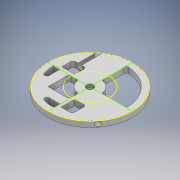
# Autodesk Inventor part: servoPlate
Saved by Autodesk Inventor 2018 (Build 220112000, 112)
## iProperties
Created: 2020-03-23
Part Number: servoPlate
Material: Generic
Document SubType Name: Modeling
Designer: technik
Density: 1 g/cm^3
Appearance: Default
Mass: 16.1735 g
Surface Area: 95.1977 cm^2
Volume: 16.1735 cm^3
Author: technik
Autodesk Inventor part; units mm, degrees
ref_plane "YZ Plane" through (0, 0, 0) normal (1, 0, 0) x (0, 1, 0)
ref_plane "XZ Plane" through (0, 0, 0) normal (0, 1, 0) x (-1, 0, 0)
ref_plane "XY Plane" through (0, 0, 0) normal (0, 0, 1) x (1, 0, 0)
sketch "Sketch1" plane through (0, 0, 0) normal (0, 0, 1) x (1, 0, 0)
  circle A0 centre (0, 0) radius 37
  dimension "d0" = 74
  constraints: 1 centre point, 1 coincident
  measures "d0" diameter of A0
extrude "Extrusion1" add sketch "Sketch1" along normal blind 5
sketch "Sketch2" plane through (0, 0, 5) normal (0, 0, 1) x (1, 0, 0)
  circle A0 centre (0, 0) radius 3
  dimension "d3" = 6
  constraints: 1 centre point, 1 coincident
  measures "d3" diameter of A0
extrude "Extrusion2" cut sketch "Sketch2" against normal blind 3
sketch "Sketch5" plane through (0, 0, 2) normal (0, 0, 1) x (1, 0, 0)
  circle A0 centre (0, 0) radius 1.75
  dimension "d6" = 3.5
  constraints: 1 centre point, 1 coincident
  measures "d6" diameter of A0
extrude "Extrusion3" cut sketch "Sketch5" along normal through all both and the other way through all
sketch "Sketch6" plane through (0, 0, 5) normal (0, 0, 1) x (1, 0, 0)
  circle A0 centre (0, 0) radius 37 projected
  line L0 (0, 37) -> (0, -37)
  line L1 (-37, 0) -> (37, 0)
  constraints: 4 end point, 4 point on circle, 1 perpendicular, 1 vertical
sketch "Sketch12" plane through (0, 0, 5) normal (0, 0, 1) x (1, 0, 0)
  ellipse E0 centre (-0.0097, 0.019) end of major axis (15.8068, 5.5327) minor radius 16.75 projected
  point P0 (0, 0)
  constraints: 1 other
sketch "Sketch13" plane through (0, 0, 5) normal (0, 0, 1) x (1, 0, 0)
  ellipse E0 centre (6.7485, -22.3457) end of major axis (6.7485, -16.3457) minor radius 0.0028 (6.7485, -28.3457) -> (6.7485, -16.3457) ccw
  line L0 (6.7485, -16.3457) -> (6.756, -16.3457)
  ellipse E1 centre (6.756, -17.3457) end of major axis (6.756, -16.3457) minor radius 0.0005 (6.7565, -17.3457) -> (6.756, -16.3457) ccw
  line L1 (6.7565, -17.3457) -> (6.7565, -27.3457)
  ellipse E2 centre (6.756, -27.3457) end of major axis (6.756, -26.3457) minor radius 0.0005 (6.756, -28.3457) -> (6.7565, -27.3457) ccw
  line L2 (6.756, -28.3457) -> (6.7485, -28.3457)
  line L3 (2.7586, -17.3457) -> (2.7586, -27.3457)
  line L4 (4.7586, -27.3457) -> (4.7586, -17.3457)
  ellipse E3 centre (2.744, -17.3457) end of major axis (2.744, -16.3457) minor radius 0.0005 (2.744, -16.3457) -> (2.7435, -17.3457) ccw
  line L5 (2.7435, -17.3457) -> (2.7435, -27.3457)
  ellipse E4 centre (2.744, -27.3457) end of major axis (2.744, -26.3457) minor radius 0.0005 (2.7435, -27.3457) -> (2.744, -28.3457) ccw
  line L6 (2.744, -28.3457) -> (2.7461, -28.3457)
  ellipse E5 centre (2.7461, -27.3457) end of major axis (2.7461, -26.3457) minor radius 0.0005 (2.7456, -27.3457) -> (2.7461, -28.3457) ccw
  line L7 (2.7456, -17.3457) -> (2.7456, -27.3457)
  ellipse E6 centre (2.7461, -17.3457) end of major axis (2.7461, -16.3457) minor radius 0.0005 (2.7461, -16.3457) -> (2.7456, -17.3457) ccw
  line L8 (2.7461, -16.3457) -> (2.744, -16.3457)
  ellipse E7 centre (2.7442, -22.3457) end of major axis (2.7442, -21.3457) minor radius 0.0005
  ellipse E8 centre (-21.634, 6.7452) end of major axis (-27.634, 6.7452) minor radius 0.0082 (-27.634, 6.7452) -> (-15.634, 6.7452) ccw
  line L9 (-27.634, 6.7452) -> (-27.634, 6.7234)
  ellipse E9 centre (-26.634, 6.7234) end of major axis (-27.634, 6.7234) minor radius 0.0014 (-27.634, 6.7234) -> (-26.634, 6.7221) ccw
  line L10 (-26.634, 6.7221) -> (-16.634, 6.722)
  ellipse E10 centre (-16.634, 6.7234) end of major axis (-17.634, 6.7234) minor radius 0.0014 (-16.634, 6.722) -> (-15.634, 6.7234) ccw
  line L11 (-15.634, 6.7234) -> (-15.634, 6.7452)
  ellipse E11 centre (-21.634, 4.7574) end of major axis (-22.634, 4.7574) minor radius 0.0014
  ellipse E12 centre (-26.634, 4.7581) end of major axis (-25.634, 4.7581) minor radius 0.0014 (-26.634, 4.7594) -> (-27.634, 4.7581) ccw
  line L12 (-27.634, 4.7581) -> (-27.634, 4.752)
  ellipse E13 centre (-26.634, 4.752) end of major axis (-25.634, 4.752) minor radius 0.0014 (-26.634, 4.7533) -> (-27.634, 4.752) ccw
  line L13 (-16.634, 4.7533) -> (-26.634, 4.7533)
  ellipse E14 centre (-16.634, 4.752) end of major axis (-15.634, 4.752) minor radius 0.0014 (-15.634, 4.752) -> (-16.634, 4.7533) ccw
  line L14 (-15.634, 4.752) -> (-15.634, 4.7581)
  ellipse E15 centre (-16.634, 4.7581) end of major axis (-15.634, 4.7581) minor radius 0.0014 (-15.634, 4.7581) -> (-16.634, 4.7594) ccw
  line L15 (-16.634, 4.7594) -> (-26.634, 4.7594)
  ellipse E16 centre (-26.634, 2.7581) end of major axis (-27.634, 2.7581) minor radius 0.0014 (-26.634, 2.7594) -> (-27.634, 2.7581) ccw
  line L16 (-26.634, 2.7594) -> (-16.634, 2.7594)
  ellipse E17 centre (-16.634, 2.7581) end of major axis (-17.634, 2.7581) minor radius 0.0014 (-15.634, 2.7581) -> (-16.634, 2.7594) ccw
  line L17 (-15.634, 2.7581) -> (-15.634, 2.752)
  ellipse E18 centre (-16.634, 2.752) end of major axis (-17.634, 2.752) minor radius 0.0014 (-15.634, 2.752) -> (-16.634, 2.7533) ccw
  line L18 (-26.634, 2.7533) -> (-16.634, 2.7533)
  ellipse E19 centre (-26.634, 2.752) end of major axis (-27.634, 2.752) minor radius 0.0014 (-26.634, 2.7533) -> (-27.634, 2.752) ccw
  line L19 (-27.634, 2.752) -> (-27.634, 2.7581)
  ellipse E20 centre (-21.634, 2.7574) end of major axis (-22.634, 2.7574) minor radius 0.0014
  line L20 (2.7461, -28.3457) -> (4.7586, -28.3457)
  line L21 (4.7586, -28.3457) -> (4.7586, -16.3457)
  line L22 (4.7586, -16.3457) -> (2.7461, -16.3457)
  line L23 (2.7461, -16.3457) -> (2.7461, -28.3457)
  line L24 (4.7586, -28.3457) -> (12.7435, -28.3457)
  line L25 (12.7435, -28.3457) -> (12.7435, -16.3457)
  line L26 (12.7435, -16.3457) -> (4.7586, -16.3457)
  line L27 (4.7586, -16.3457) -> (4.7586, -28.3457)
  line L28 (-27.634, 2.752) -> (-16.1272, 2.752)
  line L29 (-16.1272, 2.752) -> (-16.1272, 12.752)
  line L30 (-16.1272, 12.752) -> (-27.634, 12.752)
  line L31 (-27.634, 12.752) -> (-27.634, 2.752)
  point P0 (0, 0)
extrude "Extrusion9" cut sketch "Sketch13" against normal through all contours L24 L21 L4 L26 E0 | E7 | E2 L1 E1 L26 L25 L24 | L20 E4 L5 E3 L22 L21 L4 | L31 L30 L29 E8 | E8 L29 E10 L10 E9 L9 | E9 L10 E10 L29 E15 L15 E12 L31 | E12 L15 E15 L29 E14 L13 E13 L12 | E13 L13 E14 L29 E17 L16 E16 L31 | L29 E18 L18 L16 E17
sketch "Sketch14" plane through (0, 0, 5) normal (0, 0, 1) x (1, 0, 0)
  line L0 (12.7435, -16.3457) -> (12.7435, -28.3457) projected
  line L1 (2.7461, -28.3457) -> (2.7461, -16.3457) projected
  line L2 (12.7435, -16.3457) -> (2.7461, -16.3457)
  line L3 (2.7461, -16.3457) -> (2.7461, -28.3457)
  line L4 (2.7461, -28.3457) -> (12.7435, -28.3457)
  line L5 (12.7435, -28.3457) -> (12.7435, -16.3457)
  point P0 (0, 0)
  constraints: 8 end point, 2 parallel, 1 horizontal, 1 perpendicular
extrude "Extrusion10" cut sketch "Sketch14" against normal through all
sketch "Sketch17" plane through (2.7461, -28.3457, 5) normal (1, 0, 0) x (0, 0, -1)
  ellipse E0 centre (2.2619, 6) end of major axis (2.2619, 7) minor radius 1 projected
  circle A0 centre (2.2619, 6) radius 2
  point P0 (5, 28.3457)
  dimension "d47" = 4
  constraints: 1 centre point, 1 coincident, 1 other
  measures "d47" diameter of A0
extrude "Extrusion12" cut sketch "Sketch17" along normal through all contours E0 | A0
sketch "Sketch19" plane through (-27.634, 2.752, 5) normal (0, 1, 0) x (1, 0, 0)
  ellipse E0 centre (6, 1.9244) end of major axis (5, 1.924) minor radius 1 projected
  circle A0 centre (6, 1.9244) radius 2.5
  point P0 (27.634, 5)
  dimension "d52" = 5
  constraints: 1 centre point, 1 coincident, 1 other
  measures "d52" diameter of A0
extrude "Extrusion14" cut sketch "Sketch19" along normal through all contours E0 | A0
sketch "Sketch20" plane through (0, 0, 5) normal (0, 0, 1) x (1, 0, 0)
  circle A0 centre (0, 0) radius 1.75 projected
  circle A1 centre (0, 0) radius 37
  line L0 (0, 0) -> (1.75, 0)
  line L1 (10, 0) -> (32, 0)
  line L2 (0, 0) -> (0, 1.75)
  line L3 (0, 10) -> (0, 32)
  line L4 (0, 0) -> (-1.75, 0)
  line L5 (-10, 0) -> (-32, 0)
  line L6 (0, 0) -> (0, -1.75)
  line L7 (0, -10) -> (0, -32)
  arc A2 (32, 0) -> (0, 32) centre (0, 0) ccw
  arc A3 (-32, 0) -> (0, -32) centre (0, 0) ccw
  arc A4 (-10, 0) -> (0, -10) centre (0, 0) ccw
  arc A5 (10, 0) -> (0, 10) centre (0, 0) ccw
  constraints: 16 end point, 12 point on circle, 8 perpendicular, 5 centre point, 2 coincident, 2 horizontal, 2 vertical
extrude "Extrusion15" cut sketch "Sketch20" against normal blind 10 contours A5 L3 A2 L1 | A4 L7 A3 L5
sketch "Sketch21" plane through (0, 0, 5) normal (0, 0, 1) x (1, 0, 0)
  line L0 (-32, 0) -> (-10, 0) projected
  line L1 (-18.4966, 0) -> (-26.4966, 0)
  line L2 (-26.4966, 0) -> (-26.4966, -23.9158)
  line L3 (-26.4966, -23.9158) -> (-18.4966, -23.9158)
  line L4 (-18.4966, -23.9158) -> (-18.4966, 0)
  line L5 (0, -32) -> (0, -10) projected
  line L6 (0, -18.429) -> (-23.9027, -18.429)
  line L7 (-23.9027, -18.429) -> (-23.9027, -26.429)
  line L8 (-23.9027, -26.429) -> (0, -26.429)
  line L9 (0, -26.429) -> (0, -18.429)
  point P0 (0, 0)
  dimension "d59" = 8
  dimension "d60" = 8
  constraints: 16 end point, 4 parallel, 2 horizontal, 2 perpendicular, 2 point on line
  measures "d59" distance between parallel lines of L8 L6
  measures "d60" distance of L2.end L3.end
extrude "Extrusion16" add sketch "Sketch21" against normal up to surface (5 mm away)
sketch "Sketch18" plane through (-27.634, 2.752, 5) normal (0, 1, 0) x (1, 0, 0)
  ellipse E0 centre (6, 1.9244) end of major axis (5, 1.924) minor radius 1 projected
  circle A0 centre (6, 1.9244) radius 1
  point P0 (27.634, 5)
  constraints: 1 centre point, 1 coincident, 2 other
extrude "Extrusion13" cut sketch "Sketch18" against normal blind 10
sketch "Sketch15" plane through (2.7461, -28.3457, 5) normal (1, 0, 0) x (0, 0, -1)
  ellipse E0 centre (2.2619, 6) end of major axis (2.2619, 7) minor radius 1 projected
  circle A0 centre (2.2619, 6) radius 1
  point P0 (5, 28.3457)
  constraints: 1 centre point, 1 coincident, 2 other
extrude "Extrusion11" cut sketch "Sketch15" against normal blind 10
fillet "Fillet4" radius 2 9 edges at (0, -10, 2.5) (-10, 0, 2.5) (0, -18.429, 2.5) (-18.4966, 0, 2.5) (-16.1272, 12.752, 2.5) (-27.634, 12.752, 2.5) (12.7435, -16.3457, 2.5) (12.7435, -28.3457, 2.5) (0, -32, 2.5)
fillet "Fillet5" radius 2 2 edges at (-18.0419, -26.429, 2.5) (-26.4966, -17.9424, 2.5)
fillet "Fillet6" radius 2 4 edges at (32, 0, 2.5) (0, 32, 2.5) (0, 10, 2.5) (10, 0, 2.5)
body "Solid1"
